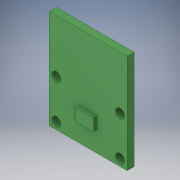
# Autodesk Inventor part: angle hall sensor
Saved by Autodesk Inventor 2019 (Build 230136000, 136)
## iProperties
Created: 2018-08-27
Part Number: angle hall sensor
Material: Generic
Document SubType Name: Modeling
Designer: Brian
Density: 1 g/cm^3
Appearance: Smooth - Dark Forest Green
Author: Brian
Autodesk Inventor part; units mm, degrees
ref_plane "YZ Plane" through (0, 0, 0) normal (1, 0, 0) x (0, 1, 0)
ref_plane "XZ Plane" through (0, 0, 0) normal (0, 1, 0) x (-1, 0, 0)
ref_plane "XY Plane" through (0, 0, 0) normal (0, 0, 1) x (1, 0, 0)
sketch "Sketch1" plane through (0, 0, 0) normal (0, 0, 1) x (1, 0, 0)
  line L0 (0, 0) -> (22, 0)
  line L1 (22, 0) -> (22, 28)
  line L2 (22, 28) -> (0, 28)
  line L3 (0, 28) -> (0, 0)
  dimension "d0" = 22
  dimension "d1" = 28
  constraints: 8 end point, 2 parallel, 1 horizontal, 1 perpendicular
  measures "d0" distance of L2.end L1.end
  measures "d1" distance of L1.end L0.end
extrude "Extrusion1" add sketch "Sketch1" along normal blind 2
sketch "Sketch2" plane through (0, 0, 2) normal (0, 0, 1) x (1, 0, 0)
  line L0 (0, 0) -> (22, 0) projected
  line L1 (0, 28) -> (0, 0) projected
  point P0 (2, 2)
  dimension "d34" = 2
  dimension "d35" = 2
  measures "d34" distance from line of L0 point (2, 2)
  measures "d35" distance from line of L1 point (2, 2)
hole "Hole1" at (2, 2, 2) direction (0, 0, -1) diameter 2.6 end through all
sketch "Sketch3" plane through (0, 0, 2) normal (0, 0, 1) x (1, 0, 0)
  line L0 (22, 0) -> (22, 28) projected
  line L1 (0, 0) -> (22, 0) projected
  point P0 (20, 2)
  dimension "d32" = 2
  dimension "d33" = 2
  measures "d32" distance from line of L0 point (20, 2)
  measures "d33" distance from line of L1 point (20, 2)
hole "Hole2" at (20, 2, 2) direction (0, 0, -1) diameter 2.6 end through all
sketch "Sketch4" plane through (0, 0, 2) normal (0, 0, 1) x (1, 0, 0)
  circle A0 centre (2, 2) radius 1.3 projected
  line L0 (0, 28) -> (0, 0) projected
  point P0 (2, 13)
  dimension "d38" = 11
  dimension "d39" = 2
  measures "d38" distance of A0.centre point (2, 13)
  measures "d39" distance from line of L0 point (2, 13)
hole "Hole3" at (2, 13, 2) direction (0, 0, -1) diameter 2.6 end through all
sketch "Sketch5" plane through (0, 0, 2) normal (0, 0, 1) x (1, 0, 0)
  line L0 (22, 0) -> (22, 28) projected
  circle A0 centre (20, 2) radius 1.3 projected
  point P0 (0, 0)
  point P1 (20, 13)
  dimension "d36" = 2
  dimension "d37" = 11
  measures "d36" distance from line of L0 point (20, 13)
  measures "d37" distance of A0.centre point (20, 13)
hole "Hole4" at (20, 13, 2) direction (0, 0, -1) diameter 2.6 end through all
sketch "Sketch6" plane through (0, 0, 2) normal (0, 0, 1) x (1, 0, 0)
  line L0 (8.5, 9.25) -> (13.5, 9.25)
  line L1 (13.5, 9.25) -> (13.5, 5.75)
  line L2 (13.5, 5.75) -> (8.5, 5.75)
  line L3 (8.5, 5.75) -> (8.5, 9.25)
  line L4 (0, 0) -> (22, 0) projected
  line L5 (0, 28) -> (0, 0) projected
  dimension "d40" = 5
  dimension "d41" = 3.5
  dimension "d42" = 5.75
  dimension "d43" = 8.5
  constraints: 8 end point, 2 parallel, 1 horizontal, 1 perpendicular
  measures "d40" distance of L1.end L2.end
  measures "d41" distance of L0.end L1.end
  measures "d42" distance between parallel lines of L4 L2
  measures "d43" distance between parallel lines of L5 L3
extrude "Extrusion2" add sketch "Sketch6" along normal blind 1
body "Solid1"
